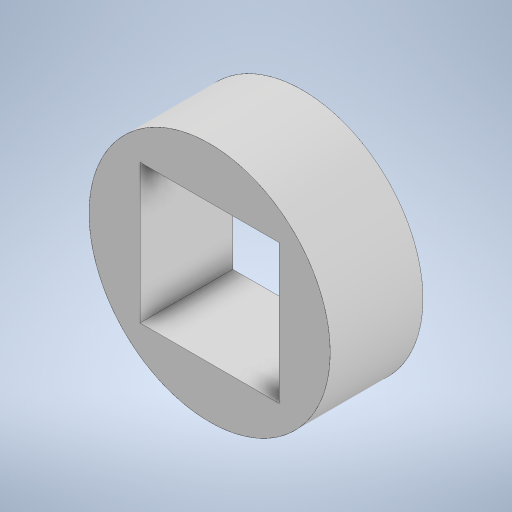
# Autodesk Inventor part: bushings
Saved by Autodesk Inventor 2023 (Build 270158000, 158)
## iProperties
Created: 2023-11-28
Part Number: bushings
Material: Generic
Document SubType Name: Modeling
Designer: Nate
Density: 1 g/cm^3
Appearance: Default
Author: Nate
Autodesk Inventor part; units mm, degrees
ref_plane "YZ Plane" through (0, 0, 0) normal (1, 0, 0) x (0, 1, 0)
ref_plane "XZ Plane" through (0, 0, 0) normal (0, 1, 0) x (-1, 0, 0)
ref_plane "XY Plane" through (0, 0, 0) normal (0, 0, 1) x (1, 0, 0)
sketch "Sketch1" plane through (0, 0, 0) normal (0, 0, 1) x (1, 0, 0)
  circle A0 centre (0, 0) radius 4.1275
  line L0 (-2.3813, 2.3813) -> (2.3812, 2.3813)
  line L1 (2.3812, 2.3813) -> (2.3812, -2.3812)
  line L2 (2.3812, -2.3812) -> (-2.3813, -2.3812)
  line L3 (-2.3813, -2.3812) -> (-2.3813, 2.3813)
  line L4 (-2.3813, 2.3813) -> (2.3812, -2.3812) construction
  line L5 (2.3812, 2.3813) -> (-2.3813, -2.3812) construction
  dimension "d0" = 8.255
  dimension "d1" = 4.7625
  dimension "d2" = 4.7625
  constraints: 12 end point, 2 midpoint, 2 parallel, 1 centre point, 1 coincident, 1 horizontal, 1 perpendicular
  measures "d0" diameter of A0
  measures "d1" distance of L1.end L2.end
  measures "d2" distance of L0.end L1.end
extrude "Extrusion1" add sketch "Sketch1" along normal blind 3.175
body "Solid1"
